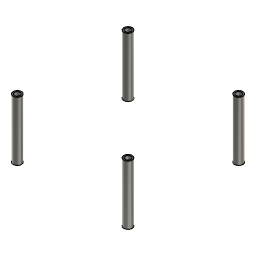
drone_assemblyfile v47 (Autodesk Fusion 360 archive; units mm, degrees)
design "Drone_BodyStandoffs"
Autodesk Fusion 360 part; units mm, degrees
sketch "Sketch1" plane through (0, 0, 0) normal (0, 0, 1) x (1, 0, 0)
  line L0 (0, 0) -> (29.9997, 29.9997)
  line L1 (0, 0) -> (42.426, 0) construction
  circle A0 centre (29.9997, 29.9997) radius 2.25
  circle A1 centre (29.9997, -29.9997) radius 2.25
  line L2 (0, 0) -> (0, 45)
  circle A2 centre (-29.9997, 29.9997) radius 2.25
  circle A3 centre (-29.9997, -29.9997) radius 2.25
  dimension "d1" = 42.426
  dimension "d2" = 45
  dimension "d3" = 4.5
  constraint horizontal L1
  constraint coincident L0.start L1.start
  constraint coincident L0.end A0.centre
  constraint symmetric L1 A0 A1
  constraint perpendicular L1 L2
  constraint symmetric A0 L2 A2
  constraint symmetric A1 L2 A3
  measures "d1" distance of L0.start L0.end
  measures "d2" angle of L0 L1
  measures "d3" diameter of A0
extrude "Extrude1" add sketch "Sketch1" along normal blind 40 makes body 1 at (-27.7525, 29.8876, 26.6667) makes body 2 at (-27.7525, -30.1119, 26.6667) makes body 3 at (32.2385, 30.2237, 26.6667) makes body 4 at (32.2469, -30.1119, 26.6667)
extrude "Extrude2" cut 4 faces at (-31.2583, 30.3025, 40) (30.6527, 30.6433, 40) (-31.0353, -29.6803, 40) (29.6247, -30.6492, 40) along direction (0, 0, -1) blind 8 on bodies 1 2 3 4 bodies 1 2 3 4
hole "Hole1" at (-29.9997, 29.9997, 32) direction (0, 0, -1) diameter 3 depth 7 tip angle 118 bodies 1
hole "Hole2" at (29.9997, 29.9997, 32) direction (0, 0, -1) diameter 3 depth 7 tip angle 118 bodies 3
hole "Hole3" at (29.9997, -29.9997, 32) direction (0, 0, -1) diameter 3 depth 7 tip angle 118 bodies 4
hole "Hole4" at (-29.9997, -29.9997, 32) direction (0, 0, -1) diameter 3 depth 7 tip angle 118 bodies 2
hole "Hole5" at (-29.9997, -29.9997, 0) direction (0, 0, 1) diameter 3 depth 7 tip angle 118 bodies 2
hole "Hole6" at (29.9997, -29.9997, 0) direction (0, 0, 1) diameter 3 depth 7 tip angle 118 bodies 4
hole "Hole7" at (29.9997, 29.9997, 0) direction (0, 0, 1) diameter 3 depth 7 tip angle 118 bodies 3
hole "Hole8" at (-29.9997, 29.9997, 0) direction (0, 0, 1) diameter 3 depth 7 tip angle 118 bodies 1
sketch "Sketch2" plane through (0, 0, 0) normal (0, 0, 1) x (1, 0, 0)
  circle A0 centre (0, 0) radius 1.75
  dimension "d33" = 3.5
  constraint coincident A0.centre origin
  measures "d33" diameter of A0
